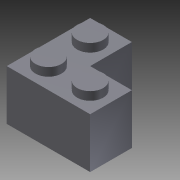
# Autodesk Inventor part: 2357
Saved by Autodesk Inventor 2011 SP1 (Build 150282100, 282)
## iProperties
Company: Allseas Engineering BV
Created: 2011-09-29
Part Number: 2357
Cost Center: 0 kg
Material: Steel
Document SubType Name: Modeling
Designer: PMe
Authority: 0 mm^3
Stock Number: =<Filenr>_<Document number>
Density: 7.85 g/cm^3
Act. Code: DW000
SaveDate: 2011-07-28
SaveTime: 18:32
FileName: Standard
TotalMass: 0 kg
TotalVolume: 0 mm^3
Subject: =<Title><TITLE 1_2> <TITLE 2_2>
Author: PMe
Autodesk Inventor part; units mm, degrees
ref_plane "YZ Plane" through (0, 0, 0) normal (1, 0, 0) x (0, 1, 0)
ref_plane "XZ Plane" through (0, 0, 0) normal (0, 1, 0) x (-1, 0, 0)
ref_plane "XY Plane" through (0, 0, 0) normal (0, 0, 1) x (1, 0, 0)
sketch "Sketch1" plane through (0, 0, 0) normal (0, 0, 1) x (1, 0, 0)
  line L0 (0, 0) -> (16, 0)
  line L1 (16, 0) -> (16, 8)
  line L2 (16, 8) -> (8, 8)
  line L3 (8, 8) -> (8, 16)
  line L4 (8, 16) -> (0, 16)
  line L5 (0, 16) -> (0, 0)
  dimension "d0" = 16
  dimension "d1" = 16
  dimension "d2" = 8
  dimension "d3" = 8
  constraints: 12 end point, 4 parallel, 1 horizontal, 1 perpendicular
  measures "d0" distance of L4.end L0.start
  measures "d1" distance of L0.start L0.end
  measures "d2" distance of L0.end L1.end
  measures "d3" distance of L3.end L4.end
extrude "Extrusion1" add sketch "Sketch1" along normal blind 9.6
sketch "Sketch2" plane through (0, 0, 9.6) normal (0, 0, 1) x (1, 0, 0)
  line L0 (16, 8) -> (16, 0) projected
  line L1 (8, 8) -> (16, 8) projected
  line L2 (8, 16) -> (8, 8) projected
  line L3 (0, 16) -> (8, 16) projected
  circle A0 centre (4, 12) radius 2.5
  circle A1 centre (4, 4) radius 2.5
  circle A2 centre (12, 4) radius 2.5
  point P0 (4, 16)
  point P1 (16, 4)
  point P2 (8, 12)
  point P3 (12, 8)
  dimension "d6" = 5
  constraints: 4 midpoint, 3 centre point, 3 horizontal alignment, 3 vertical alignment, 2 equal radius
  measures "d6" diameter of A1
extrude "Extrusion2" add sketch "Sketch2" along normal blind 1.6
shell "Shell1" thickness 1.5 removed faces 1 at (2.6667, 8, 0)
equation "\"d0\" = d1"
equation "\"d2\" = 0.5 * d1"
equation "\"d3\" = d2"
body "Solid1"
